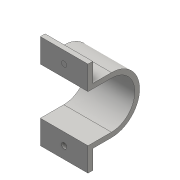
# Autodesk Inventor part: Motor mount
Saved by Autodesk Inventor 2016 (Build 200138000, 138)
## iProperties
Created: 2016-04-05
Part Number: Motor mount
Material: Generic
Document SubType Name: Modeling
Designer: Ariana
Density: 1 g/cm^3
Appearance: Default
Author: Ariana
Autodesk Inventor part; units mm, degrees
ref_plane "YZ Plane" through (0, 0, 0) normal (1, 0, 0) x (0, 1, 0)
ref_plane "XZ Plane" through (0, 0, 0) normal (0, 1, 0) x (-1, 0, 0)
ref_plane "XY Plane" through (0, 0, 0) normal (0, 0, 1) x (1, 0, 0)
sketch "Sketch1" plane through (0, 0, 0) normal (1, 0, 0) x (0, 1, 0)
  arc A0 (0, -12.5) -> (0, 12.5) centre (0, 0) ccw
  line L0 (-12.5, -25.2) -> (-9.96, -25.2)
  line L1 (-9.96, -25.2) -> (-9.96, -15.04)
  line L2 (-12.5064, 25.2) -> (-9.9664, 25.2)
  line L3 (-12.5064, 25.2) -> (-12.5064, 12.5)
  line L4 (-12.5, -12.5) -> (-12.5, -25.2)
  line L5 (-9.9664, 15.04) -> (-9.9664, 25.2)
  arc A1 (0, -15.04) -> (0, 15.04) centre (0, 0) ccw
  line L6 (0, 15.04) -> (-9.9664, 15.04)
  line L7 (0, 12.5) -> (-12.5064, 12.5)
  line L8 (0, -12.5) -> (-12.5, -12.5)
  line L9 (0, -15.04) -> (-9.96, -15.04)
  point P0 (-4.98, -15)
  dimension "d0" = 25
  dimension "d9" = 12.7
  dimension "d10" = 12.7
  dimension "d11" = 2.54
  dimension "d12" = 2.54
  dimension "d15" = 2.54
  dimension "d17" = 0.0064
  dimension "d23" = 0
  dimension "d24" = 0
  dimension "d25" = 0
  dimension "d26" = 0
  dimension "d27" = 0.04
  dimension "d28" = 4.98
  constraints: 20 end point, 4 perpendicular, 4 point on circle, 3 parallel, 2 centre point, 2 vertical, 1 coincident, 1 horizontal, 1 tangent
  measures "d0" diameter of A0
  measures "d9" distance of L2.start L3.end
  measures "d10" distance of L4.start L0.start
  measures "d11" distance of L0.start L0.end
  measures "d12" distance of L2.start L2.end
  measures "d15" radial gap between concentric circles of A0 A1
  measures "d17" distance between parallel lines of L5 L1
  measures "d23" horizontal distance of L7.start point (0, 0)
  measures "d24" horizontal distance of point (0, 0) L6.start
  measures "d25" horizontal distance of point (0, 0) L8.start
  measures "d26" horizontal distance of point (0, 0) L9.start
  measures "d27" distance from line of point (-4.98, -15) L9
  measures "d28" distance from line of point (-4.98, -15) L1
extrude "Extrusion1" add sketch "Sketch1" along normal blind 25.4
sketch "Sketch2" plane through (0, -12.5, -25.2) normal (0, -1, 0) x (1, 0, 0)
  circle A0 centre (12.7, 44.05) radius 1.4224
  circle A1 centre (12.7, 6.35) radius 1.4224
  line L0 (0, 50.4) -> (25.4, 50.4) projected
  line L1 (25.4, 50.4) -> (25.4, 37.7) projected
  line L2 (0, 0) -> (25.4, 0) projected
  point P0 (0, 25.2)
  dimension "d31" = 2.8448
  dimension "d32" = 6.35
  dimension "d33" = 12.7
  dimension "d34" = 0
  dimension "d35" = 6.35
  dimension "d36" = 2.8448
  constraints: 2 centre point
  measures "d31" diameter of A0
  measures "d32" distance from line of L0 A0.centre
  measures "d33" distance from line of L1 A0.centre
  measures "d34" horizontal distance of A0.centre A1.centre
  measures "d35" distance from line of L2 A1.centre
  measures "d36" diameter of A1
extrude "Extrusion2" cut sketch "Sketch2" against normal blind 25.4
body "Solid1"
